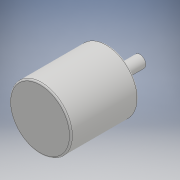
# Autodesk Inventor part: IG42C-144
Saved by Autodesk Inventor 2017 (Build 210142000, 142)
## iProperties
Part Number: IG42C-144
Material: 一般
Document SubType Name: Modeling
Designer: highs
Density: 1 g/cm^3
Appearance: 既定
Author: highs
Autodesk Inventor part; units mm, degrees
ref_plane "YZ Plane" through (0, 0, 0) normal (1, 0, 0) x (0, 1, 0)
ref_plane "XZ Plane" through (0, 0, 0) normal (0, 1, 0) x (-1, 0, 0)
ref_plane "XY Plane" through (0, 0, 0) normal (0, 0, 1) x (1, 0, 0)
sketch "スケッチ1" plane through (0, 0, 0) normal (0, 0, 1) x (1, 0, 0)
  line L0 (0, 0) -> (21, 0)
  line L1 (21, 0) -> (21, 45.9)
  line L2 (21, 45.9) -> (12.5, 45.9)
  line L3 (12.5, 45.9) -> (12.5, 47.9)
  line L4 (12.5, 47.9) -> (8, 47.9)
  line L5 (8, 47.9) -> (8, 49.2)
  line L6 (8, 49.2) -> (4, 49.2)
  line L7 (4, 49.2) -> (4, 67.9)
  line L8 (4, 67.9) -> (0, 67.9)
  line L9 (0, 67.9) -> (0, 0)
  dimension "d0" = 21
  dimension "d1" = 4
  dimension "d2" = 12.5
  dimension "d3" = 2
  dimension "d4" = 8
  dimension "d5" = 1.3
  dimension "d6" = 45.9
  dimension "d8" = 20
  constraints: 20 end point, 9 perpendicular, 1 horizontal
  measures "d0" distance of L0.start L0.end
  measures "d1" distance of L7.end L8.end
  measures "d2" distance between parallel lines of L9 L3
  measures "d3" distance of L2.end L3.end
  measures "d4" distance between parallel lines of L9 L5
  measures "d5" distance of L4.end L5.end
  measures "d6" distance of L0.end L1.end
  measures "d8" distance between parallel lines of L4 L8
revolve "回転1" add sketch "スケッチ1" angle 360 about axis through (0, 67.9, 0) along (0, -1, 0)
sketch "スケッチ2" plane through (0, 67.9, 0) normal (0, 1, 0) x (1, 0, 0)
  line L0 (-2.6458, 3) -> (2.6458, 3)
  circle A0 centre (0, 0) radius 4 projected
  arc A1 (2.6458, 3) -> (-2.6458, 3) centre (0, 0) ccw
  dimension "d10" = 3
  constraints: 4 point on circle, 2 end point, 1 centre point, 1 coincident, 1 horizontal
  measures "d10" distance from line of L0 point (0, 0)
extrude "押し出し1" cut sketch "スケッチ2" against normal blind 12 contours A0 L0 picked at (0.5822, 3.4764)
sketch "スケッチ4" plane through (0, 47.9, 0) normal (0, 1, 0) x (1, 0, 0)
  line L0 (0, 0) -> (0, 29.0549) construction
  arc A0 (11.5, -4.899) -> (11.5, 4.899) centre (0, 0) ccw
  line L1 (11.5, 4.899) -> (11.5, -4.899)
  circle A1 centre (0, 0) radius 12.5 projected
  arc A2 (-11.5, 4.899) -> (-11.5, -4.899) centre (0, 0) ccw
  line L2 (-11.5, 4.899) -> (-11.5, -4.899)
  dimension "d13" = 11.5
  constraints: 6 end point, 4 point on circle, 2 centre point, 2 symmetric about line, 2 vertical, 1 coincident, 3 other
  measures "d13" distance between parallel lines of L1 L0
extrude "押し出し2" cut sketch "スケッチ4" against normal blind 2 contours L1 A0 | A1 L2
fillet "フィレット1" radius 1 2 edges at (-21, 45.9, 0) (-21, 0, 0)
sketch "スケッチ5" plane through (0, 45.9, 0) normal (0, 1, 0) x (1, 0, 0)
  circle A0 centre (0, 0) radius 17.5 construction
  circle A1 centre (-17.5, 0) radius 1.75
  line L0 (0, 0) -> (-17.5, 0) construction
  circle A2 centre (0, -17.5) radius 1.75
  circle A3 centre (17.5, 0) radius 1.75
  circle A4 centre (0, 17.5) radius 1.75
  dimension "d18" = 35
  dimension "d17" = 3.5
  dimension "d21" = 360
  constraints: 4 centre point, 2 end point, 1 coincident, 1 horizontal, 1 horizontal alignment, 11 other
  measures "d17" diameter of A1
extrude "押し出し3" cut sketch "スケッチ5" against normal blind 5
